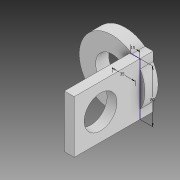
# Autodesk Inventor part: Wrist
Saved by Autodesk Inventor 2020 (Build 240168000, 168)
## iProperties
Created: 2021-03-19
Part Number: Wrist
Material: Generic
Document SubType Name: Modeling
Designer: DDeGo
Density: 1 g/cm^3
Appearance: Default
Author: DDeGo
Autodesk Inventor part; units mm, degrees
ref_plane "YZ Plane" through (0, 0, 0) normal (1, 0, 0) x (0, 1, 0)
ref_plane "XZ Plane" through (0, 0, 0) normal (0, 1, 0) x (-1, 0, 0)
ref_plane "XY Plane" through (0, 0, 0) normal (0, 0, 1) x (1, 0, 0)
sketch "Sketch1" plane through (0, 0, 0) normal (0, 0, 1) x (1, 0, 0)
  circle A0 centre (0, 0) radius 50
  circle A1 centre (0, 0) radius 25
  dimension "d0" = 50
  dimension "d1" = 100
  constraints: 2 centre point, 2 coincident
  measures "d0" diameter of A1
  measures "d1" diameter of A0
extrude "Extrusion1" add sketch "Sketch1" along normal blind 20
sketch "Sketch2" plane through (0, 0, 20) normal (0, 0, 1) x (1, 0, 0)
  line L0 (27.5, -40) -> (42.5, -40)
  line L1 (42.5, -40) -> (42.5, 40)
  line L2 (42.5, 40) -> (27.5, 40)
  line L3 (27.5, 40) -> (27.5, -40)
  line L4 (27.5, -40) -> (42.5, 40) construction
  line L5 (42.5, -40) -> (27.5, 40) construction
  line L6 (0, 0) -> (35, 0) construction
  dimension "d4" = 15
  dimension "d5" = 80
  dimension "d6" = 35
  constraints: 14 end point, 2 horizontal, 2 midpoint, 2 parallel, 1 perpendicular
  measures "d4" distance of L1.end L2.end
  measures "d5" distance of L0.end L1.end
  measures "d6" distance of L6.start L6.end
extrude "Extrusion2" add sketch "Sketch2" against normal up to surface (20 mm away)
extrude "Extrusion3" add sketch "Sketch2" along normal blind 100
sketch "Sketch3" plane through (27.5, -40, 20) normal (-1, 0, 0) x (0, 0, 1)
  line L0 (100, 0) -> (100, 80) projected
  line L1 (100, 40) -> (60, 40) construction
  circle A0 centre (60, 40) radius 25
  point P0 (-20, 40)
  dimension "d11" = 50
  dimension "d12" = 40
  constraints: 2 end point, 1 centre point, 1 coincident, 1 horizontal, 1 midpoint
  measures "d11" diameter of A0
  measures "d12" distance of L1.start L1.end
extrude "Extrusion4" cut sketch "Sketch3" against normal through all
body "Solid1"
